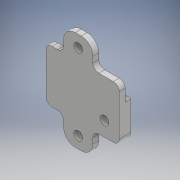
# Autodesk Inventor part: imu_MPU6050Holder_V2
Saved by Autodesk Inventor 2017 (Build 210142000, 142)
## iProperties
Created: 2017-05-21
Part Number: imu_MPU6050Holder_V2
Material: Generic
Document SubType Name: Modeling
Designer: Andi
Density: 1 g/cm^3
Appearance: Default
Author: Andi
Autodesk Inventor part; units mm, degrees
ref_plane "YZ Plane" through (0, 0, 0) normal (1, 0, 0) x (0, 1, 0)
ref_plane "XZ Plane" through (0, 0, 0) normal (0, 1, 0) x (-1, 0, 0)
ref_plane "XY Plane" through (0, 0, 0) normal (0, 0, 1) x (1, 0, 0)
sketch "Sketch1" plane through (0, 0, 0) normal (0, 1, 0) x (-1, 0, 0)
  line L0 (0, 26) -> (0, 0)
  line L1 (0, 9) -> (6, 9)
  line L2 (6, 9) -> (-9, 9)
  line L3 (11, 6) -> (11, 16)
  line L4 (-14, 16) -> (-14, 6)
  line L5 (1, 30) -> (-1, 30)
  line L6 (-1, -4) -> (1, -4)
  arc A0 (5, 26) -> (1, 30) centre (1, 26) ccw
  arc A1 (-1, 30) -> (-5, 26) centre (-1, 26) ccw
  arc A2 (1, -4) -> (5, 0) centre (1, 0) ccw
  arc A3 (-5, 0) -> (-1, -4) centre (-1, 0) ccw
  line L7 (7, 22) -> (9, 22)
  line L8 (9, 4) -> (7, 4)
  line L9 (-12, 4) -> (-7, 4)
  line L10 (-7, 22) -> (-12, 22)
  line L11 (-14, 20) -> (-14, 16)
  line L12 (-5, 24) -> (-5, 26)
  line L13 (-5, 2) -> (-5, 0)
  arc A4 (-7, 22) -> (-5, 24) centre (-7, 24) ccw
  arc A5 (-12, 22) -> (-14, 20) centre (-12, 20) ccw
  arc A6 (-14, 6) -> (-12, 4) centre (-12, 6) ccw
  arc A7 (-5, 2) -> (-7, 4) centre (-7, 2) ccw
  line L14 (5, 26) -> (5, 24)
  line L15 (5, 2) -> (5, 0)
  arc A8 (5, 24) -> (7, 22) centre (7, 24) ccw
  arc A9 (11, 20) -> (9, 22) centre (9, 20) ccw
  arc A10 (9, 4) -> (11, 6) centre (9, 6) ccw
  arc A11 (7, 4) -> (5, 2) centre (7, 2) ccw
  line L16 (11, 16) -> (11, 20)
  line L17 (11, 16) -> (-14, 16)
  line L18 (9, 4) -> (-12, 4)
  circle A12 centre (6, 9) radius 1.5
  point P0 (0, 0)
  point P1 (-14, 4)
  point P2 (5, 22)
  point P3 (11, 22)
  point P4 (5, 4)
  dimension "d9" = 6
  dimension "d10" = 26
  dimension "d11" = 9
  dimension "d12" = 15
  dimension "d13" = 5
  dimension "d14" = 5
  dimension "d17" = 4
  dimension "d18" = 4
  dimension "d20" = 4
  dimension "d21" = 4
  dimension "d22" = 4
  dimension "d23" = 4
  dimension "d25" = 5
  dimension "d26" = 5
  dimension "d27" = 18
  dimension "d28" = 1
  dimension "d29" = 2
  dimension "d30" = 6
  dimension "d31" = 1
  dimension "d32" = 6
  dimension "d34" = 4
  dimension "d35" = 2
  dimension "d37" = 10
  dimension "d38" = 6
  dimension "d39" = 2
  dimension "d54" = 3
  constraints: 38 end point, 24 point on circle, 21 tangent, 13 centre point, 9 equal radius, 8 point on line, 5 horizontal, 5 vertical, 3 collinear, 2 coincident, 2 parallel, 1 perpendicular
  measures "d9" distance of L1.start L1.end
  measures "d10" distance of L0.start L0.end
  measures "d11" distance from line of L0.end L1
  measures "d12" distance of L1.end L2.end
  measures "d13" horizontal distance of point (-14, 4) L2.end
  measures "d14" horizontal distance of point (-14, 4) L2.end
  measures "d17" distance from line of L5 L0.start
  measures "d18" distance from line of L6 L0.end
  measures "d20" radius of A0
  measures "d21" distance from line of L7 L14.start
  measures "d22" distance from line of L8 L15.end
  measures "d23" distance from line of L10 L12.end
  measures "d25" distance between parallel lines of L12 L0
  measures "d26" distance between parallel lines of L0 L13
  measures "d27" distance between parallel lines of L9 L10
  measures "d28" distance of A3.centre L0.end
  measures "d29" radius of A4
  measures "d30" distance of point (5, 22) point (11, 22)
  measures "d31" distance of L0.start A0.centre
  measures "d32" distance from line of L7 L3.end
  measures "d34" distance of point (5, 4) L15.end
  measures "d35" radius of A8
  measures "d37" distance of L3.start L3.end
  measures "d38" distance between parallel lines of L16 L14
  measures "d39" distance of L8.start L8.end
  measures "d54" diameter of A12
extrude "Extrusion1" add sketch "Sketch1" along normal blind 2 contours A12 | L17 L3 A10 L8 L18 L0 | L17 L11 A5 L10 A4 L12 A1 L5 A0 L14 A8 L7 A9 L16 | L0 L18 L9 A6 L4 L17 | L18 A11 L15 A2 L6 A3 L13 A7
extrude "Extrusion2" add sketch "Sketch1" along normal blind 4 contours A12 | L17 L3 A10 L8 L18 L0 | L0 L18 L9 A6 L4 L17
hole "Hole1" at (0, 0, 26) at (9, 0, 9) at (0, 0, 0) direction (0, 1, 0) diameter 3 depth 8 tip angle 118
extrude "Extrusion4" add sketch "Sketch1" along normal blind 5 contours A12
body "Solid1"
